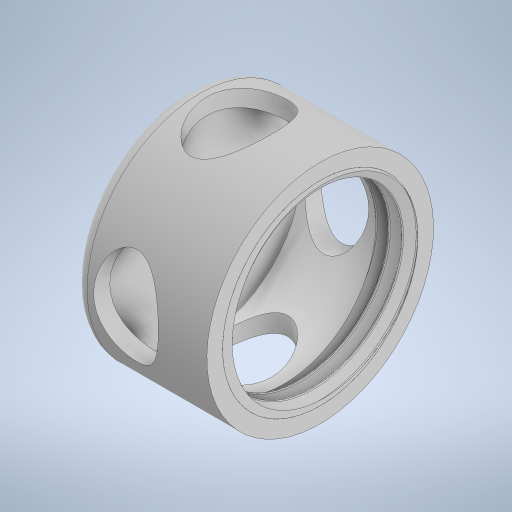
# Autodesk Inventor part: restrainer_front_electrical_magnets_2.5mm
Saved by Autodesk Inventor 2023 (Build 270158000, 158)
## iProperties
Created: 2022-11-01
Part Number: restrainer_front_electrical_magnets_2.5mm
Material: Generic
Document SubType Name: Modeling
Designer: Admin
Density: 1 g/cm^3
Appearance: Default
Author: Admin
Autodesk Inventor part; units mm, degrees
ref_plane "YZ Plane" through (0, 0, 0) normal (1, 0, 0) x (0, 1, 0)
ref_plane "XZ Plane" through (0, 0, 0) normal (0, 1, 0) x (-1, 0, 0)
ref_plane "XY Plane" through (0, 0, 0) normal (0, 0, 1) x (1, 0, 0)
sketch "Sketch1" plane through (0, 0, 0) normal (1, 0, 0) x (0, 1, 0)
  circle A0 centre (0, 0) radius 15
  circle A1 centre (0, 0) radius 17.5
  dimension "d0" = 30
  dimension "d1" = 35
  constraints: 2 centre point, 2 coincident
  measures "d0" diameter of A0
  measures "d1" diameter of A1
extrude "Extrusion2" add sketch "Sketch1" along normal blind 2.5 contours A0
sketch "Sketch2" plane through (0, 0, 0) normal (0, 1, 0) x (-1, 0, 0)
  ellipse E0 centre (-8, 0) end of major axis (-3, 0) minor radius 7.5
  line L0 (0, 15) -> (0, -15) projected
  point P0 (0, 0)
  dimension "d6" = 5
  dimension "d7" = 7.5
  dimension "d8" = 8
  constraints: 1 centre point, 1 other
  measures "d8" distance from line of L0 E0.centre
sketch "Sketch3" plane through (0, 0, 0) normal (0, 0, 1) x (1, 0, 0)
  ellipse E0 centre (8, 0) end of major axis (13, 0) minor radius 7.5
  line L0 (0, 9.8) -> (0, -9.8) projected
  point P0 (0, 0)
  dimension "d9" = 5
  dimension "d10" = 7.5
  dimension "d11" = 8
  constraints: 1 centre point, 1 other
  measures "d11" distance from line of L0 E0.centre
extrude "Extrusion3" add sketch "Sketch1" along normal blind 20.5
extrude "Extrusion4" cut sketch "Sketch3" along normal mid plane 40
extrude "Extrusion5" cut sketch "Sketch2" along normal mid plane 40
fillet "Fillet1" radius 2 1 edges at (0, -17.5, 0)
sketch "Sketch8" plane through (20.5, 0, 0) normal (1, 0, 0) x (0, 0, -1)
  circle A0 centre (0, 0) radius 15.075
  dimension "d59" = 30.15
  constraints: 1 centre point, 1 coincident
  measures "d59" diameter of A0
extrude "Extrusion7" cut sketch "Sketch8" against normal blind 5
thread "Thread6" size "M30x2" class "6H" standard "ANSI Metric M Profile" length 5
sketch "Sketch16" plane through (20.5, 0, 0) normal (0, -1, 0) x (0, 0, 1)
  line L0 (15.075, 0) -> (15.075, 5)
  line L1 (15.075, 5) -> (13.5921, 5)
  line L2 (13.5921, 5) -> (13.5921, 0)
  line L3 (13.5921, 0) -> (15.075, 0)
  line L4 (0, -6.7171) -> (0, 25.0362) projected
  constraints: 8 end point
revolve "Revolution6" add sketch "Sketch16" angle 360 about axis through (20.5, 0, 0) along (-1, 0, 0) separate body
sketch "Sketch15" plane through (20.5, 0, 15.075) normal (0, 1, 0) x (-1, 0, 0)
  line L0 (-1.1668, -0.1013) -> (-1.0001, -0.1013) construction
  line L1 (0.1666, -1.382) -> (-0.0001, -1.7021) construction
  line L2 (-2.0001, -1.7021) -> (-2.1668, -1.382) construction
  line L3 (-0.8334, -0.1013) -> (-1.0001, 0.2189) construction
  line L4 (-1.0001, 0.2189) -> (-1.1668, -0.1013) construction
  line L5 (-2.0001, -1.7021) -> (-1.8334, -1.382) construction
  line L6 (-0.8334, -0.1013) -> (-0.1668, -1.382)
  line L7 (-2.1668, -1.382) -> (-1.8334, -1.382) construction
  arc A0 (-2.1668, -1.382) -> (-2.0001, -1.4831) centre (-2.0001, -1.2952) ccw construction
  line L8 (0.1666, -1.382) -> (-0.1668, -1.382) construction
  line L9 (-2.0001, -1.7021) -> (-2.0001, -1.382) construction
  line L10 (-0.0001, -1.7021) -> (-0.0001, -1.382) construction
  line L11 (-1.0001, 0.2189) -> (-1.0001, -0.0002) construction
  line L12 (-2.0001, -1.4831) -> (-0.0001, -1.4831)
  arc A1 (-2.0001, -1.4831) -> (-1.8334, -1.382) centre (-2.0001, -1.2952) ccw
  line L13 (-0.1668, -1.382) -> (-0.0001, -1.7021) construction
  line L14 (-1.8334, -1.382) -> (-1.1668, -0.1013)
  line L15 (-0.0001, -0.0002) -> (-0.0001, 0.0177)
  line L16 (-0.0001, 0.0177) -> (-0.0001, -0.0002)
  line L17 (-0.0001, -0.0002) -> (0.0334, -0.0002)
  arc A2 (-0.1668, -1.382) -> (-0.0001, -1.4831) centre (-0.0001, -1.2952) ccw
  arc A3 (-0.0001, -1.4831) -> (0.1666, -1.382) centre (-0.0001, -1.2952) ccw construction
  arc A4 (-1.0001, -0.0002) -> (-1.1668, -0.1013) centre (-1.0001, -0.1881) ccw
  arc A5 (-0.8334, -0.1013) -> (-1.0001, -0.0002) centre (-1.0001, -0.1881) ccw
  line L18 (-1.0001, -0.0002) -> (-1.0001, -0.1013) construction
  line L19 (-1.0001, -0.1013) -> (-0.8334, -0.1013) construction
  dimension "d127" = 55
  dimension "d128" = 0.3202
  dimension "d129" = 0.3202
  dimension "Sketch15_ThreadOffset" = 0
  dimension "Sketch15_MajorRadius" = 1.4829
  dimension "d132" = 2
  dimension "Sketch15_MinorRadius" = 0
  constraints: 40 end point, 12 point on circle, 10 parallel, 8 tangent, 6 centre point, 6 collinear, 2 midpoint, 2 point on line, 1 horizontal, 1 perpendicular, 3 other
  measures "d127" angle of L6 L14
  measures "d128" distance of L3.end L0.end
  measures "d129" distance of L1.end L10.end
  measures "Sketch15_ThreadOffset" distance between parallel lines of L15 L10
  measures "Sketch15_MajorRadius" distance from line of L12 L15.start
  measures "d132" distance from line of L1.end L9
  measures "Sketch15_MinorRadius" distance edge to line of A5 L17
coil "Coil6" sketch "Sketch15" operation cut axis through (20.5, 0, 0) along (-1, 0, 0) pitch 2.002 turns 4.495504 hand right bodies 2
equation "\"d127\" = d134"
equation "\"d128\" = 0.160083 * Sketch15_Pitch"
equation "\"d129\" = 0.160083 * Sketch15_Pitch"
equation "\"d132\" = Sketch15_Pitch"
equation "\"d27\" = 55deg"
equation "\"Sketch4_Pitch\" = 2"
equation "\"d48\" = 55deg"
equation "\"Sketch6_Pitch\" = 2"
equation "\"d71\" = 55deg"
equation "\"Sketch9_Pitch\" = 2"
equation "\"d92\" = 55deg"
equation "\"Sketch11_Pitch\" = 2.5"
equation "\"d114\" = 55deg"
equation "\"Sketch13_Pitch\" = 2"
equation "\"d134\" = 55deg"
equation "\"Sketch15_Pitch\" = 2"
body "Solid1"
body "Solid7"
